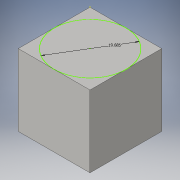
# Autodesk Inventor part: Mass
Saved by Autodesk Inventor 2016 (Build 200138000, 138)
## iProperties
Created: 2015-09-12
Part Number: Mass
Material: Generic
Document SubType Name: Modeling
Designer: nightstalker
Density: 1 g/cm^3
Appearance: Default
Mass: 8000 g
Surface Area: 2400 cm^2
Volume: 8000 cm^3
Author: nightstalker
Autodesk Inventor part; units mm, degrees
ref_plane "YZ Plane" through (0, 0, 0) normal (1, 0, 0) x (0, 1, 0)
ref_plane "XZ Plane" through (0, 0, 0) normal (0, 1, 0) x (-1, 0, 0)
ref_plane "XY Plane" through (0, 0, 0) normal (0, 0, 1) x (1, 0, 0)
sketch "Sketch4" plane through (0, 0, 0) normal (0, 0, 1) x (1, 0, 0)
  line L0 (0, 0) -> (500, 0)
  line L1 (500, 0) -> (500, 500)
  line L2 (500, 500) -> (0, 500)
  line L3 (0, 500) -> (0, 0)
  dimension "d11" = 500
  dimension "d12" = 500
  constraints: 8 end point, 2 parallel, 1 horizontal, 1 perpendicular
  measures "d11" distance of L2.end L1.end
  measures "d12" distance of L1.end L0.end
extrude "Extrusion4" add sketch "Sketch4" along normal blind 500
sketch "Sketch5" plane through (0, 500, 0) normal (0, 1, 0) x (1, 0, 0)
  circle A0 centre (250, -250) radius 250
  point P0 (0, 0)
  dimension "d15" = 500
  constraints: 1 centre point
  measures "d15" diameter of A0
body "Solid4"
